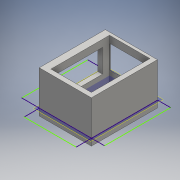
# Autodesk Inventor part: sampleHolderEnclosure
Saved by Autodesk Inventor 2016 (Build 200138000, 138)
## iProperties
Created: 2016-04-10
Part Number: sampleHolderEnclosure
Material: Generic
Document SubType Name: Modeling
Designer: sims01
Density: 1 g/cm^3
Appearance: Default
Author: sims01
Autodesk Inventor part; units mm, degrees
ref_plane "YZ Plane" through (0, 0, 0) normal (1, 0, 0) x (0, 1, 0)
ref_plane "XZ Plane" through (0, 0, 0) normal (0, 1, 0) x (-1, 0, 0)
ref_plane "XY Plane" through (0, 0, 0) normal (0, 0, 1) x (1, 0, 0)
sketch "Sketch1" plane through (0, 0, 0) normal (0, 0, 1) x (1, 0, 0)
  line L0 (-28, 35.5) -> (28, 35.5)
  line L1 (28, 35.5) -> (28, -35.5)
  line L2 (28, -35.5) -> (-28, -35.5)
  line L3 (-28, -35.5) -> (-28, 35.5)
  line L4 (-20.5, 32.5) -> (23, 32.5)
  line L5 (23, 32.5) -> (23, -30.5)
  line L6 (23, -30.5) -> (-20.5, -30.5)
  line L7 (-20.5, -30.5) -> (-20.5, 32.5)
  point P0 (0, 0)
  dimension "d0" = 56
  dimension "d1" = 28
  dimension "d2" = 71
  dimension "d3" = 35.5
  dimension "d4" = 3
  dimension "d5" = 7.5
  dimension "d7" = 5
  dimension "d8" = 5
  constraints: 16 end point, 4 parallel, 2 horizontal, 2 perpendicular
  measures "d0" distance of L0.start L0.end
  measures "d1" distance from line of point (0, 0) L1
  measures "d2" distance of L2.end L0.start
  measures "d3" distance from line of point (0, 0) L0
  measures "d4" distance between parallel lines of L4 L0
  measures "d5" distance between parallel lines of L3 L7
  measures "d7" distance between parallel lines of L2 L6
  measures "d8" distance between parallel lines of L1 L5
extrude "Extrusion1" add sketch "Sketch1" along normal blind 45
sketch "Sketch2" plane through (-28, -35.5, 0) normal (-1, 0, 0) x (0, 0, 1)
  line L0 (37.5, 60.5) -> (12.5, 60.5)
  line L1 (12.5, 60.5) -> (12.5, 10.5)
  line L2 (12.5, 10.5) -> (37.5, 10.5)
  line L3 (37.5, 10.5) -> (37.5, 60.5)
  point P0 (0, 35.5)
  dimension "d11" = 50
  dimension "d12" = 25
  dimension "d13" = 25
  dimension "d14" = 12.5
  constraints: 8 end point, 2 parallel, 1 horizontal, 1 perpendicular
  measures "d11" distance of L2.end L0.start
  measures "d12" distance from line of point (0, 35.5) L2
  measures "d13" distance of L1.end L2.end
  measures "d14" distance from line of point (0, 35.5) L1
extrude "Extrusion2" cut sketch "Sketch2" against normal up to surface (7.5 mm away)
sketch "Sketch4" plane through (-28, -35.5, 0) normal (-1, 0, 0) x (0, 0, 1)
  line L0 (40, 64.25) -> (10, 64.25)
  line L1 (10, 64.25) -> (10, 6.75)
  line L2 (10, 6.75) -> (40, 6.75)
  line L3 (40, 6.75) -> (40, 64.25)
  line L4 (0, 0) -> (0, 71) projected
  point P0 (0, 35.5)
  dimension "d23" = 57.5
  dimension "d24" = 30
  dimension "d25" = 28.75
  dimension "d26" = 10
  constraints: 8 end point, 2 parallel, 1 horizontal, 1 perpendicular
  measures "d23" distance of L2.end L0.start
  measures "d24" distance of L0.start L0.end
  measures "d25" distance from line of point (0, 35.5) L2
  measures "d26" distance between parallel lines of L4 L1
extrude "Extrusion4" cut sketch "Sketch4" against normal blind 2.5
sketch "Sketch5" plane through (-28, 35.5, 0) normal (0, 1, 0) x (1, 0, 0)
  line L0 (51.75, -40) -> (4.25, -40)
  line L1 (4.25, -40) -> (4.25, -10)
  line L2 (4.25, -10) -> (51.75, -10)
  line L3 (51.75, -10) -> (51.75, -40)
  line L4 (0, 0) -> (56, 0) projected
  point P0 (28, 0)
  dimension "d29" = 10
  dimension "d30" = 30
  dimension "d31" = 47.5
  dimension "d32" = 23.75
  constraints: 8 end point, 2 parallel, 1 horizontal, 1 perpendicular
  measures "d29" distance between parallel lines of L4 L2
  measures "d30" distance of L0.end L1.end
  measures "d31" distance of L0.start L0.end
  measures "d32" distance from line of L1 point (28, 0)
extrude "Extrusion5" cut sketch "Sketch5" against normal blind 2.5
sketch "Sketch6" plane through (-28, 35.5, 0) normal (0, 1, 0) x (1, 0, 0)
  line L0 (48, -37.5) -> (8, -37.5)
  line L1 (8, -37.5) -> (8, -12.5)
  line L2 (8, -12.5) -> (48, -12.5)
  line L3 (48, -12.5) -> (48, -37.5)
  point P0 (28, 0)
  dimension "d35" = 40
  dimension "d36" = 20
  dimension "d37" = 25
  dimension "d38" = 12.5
  constraints: 8 end point, 2 parallel, 1 horizontal, 1 perpendicular
  measures "d35" distance of L0.start L0.end
  measures "d36" distance from line of point (28, 0) L1
  measures "d37" distance of L2.end L0.start
  measures "d38" distance from line of point (28, 0) L2
extrude "Extrusion6" cut sketch "Sketch6" against normal up to surface (3 mm away)
ref_plane "Work Plane1" through (0, 0, 7.5) normal (0, 0, -1) x (-1, 0, 0)
sketch "Sketch8" plane through (0, 0, 7.5) normal (0, 0, -1) x (-1, 0, 0)
  line L0 (-42, 35.5) -> (-28, 35.5)
  line L1 (-28, 35.5) -> (-28, -35.5)
  line L2 (-28, -35.5) -> (-42, -35.5)
  line L3 (-42, -35.5) -> (-42, 35.5)
  line L4 (-28, -35.5) -> (28, -35.5)
  line L5 (28, -35.5) -> (28, -52)
  line L6 (28, -52) -> (-28, -52)
  line L7 (-28, -52) -> (-28, -35.5)
  line L8 (28, 35.5) -> (47, 35.5)
  line L9 (47, 35.5) -> (47, -35.5)
  line L10 (47, -35.5) -> (28, -35.5)
  line L11 (28, -35.5) -> (28, 35.5)
  line L12 (-28, 35.5) -> (28, 35.5) projected
  line L13 (28, -35.5) -> (-28, -35.5) projected
  line L14 (-28, -35.5) -> (-28, 35.5) projected
  line L15 (28, 35.5) -> (28, -35.5) projected
  point P0 (0, 0)
  constraints: 24 end point, 9 collinear, 6 parallel, 3 horizontal, 3 perpendicular
equation "\"d1\" = 0.5 * d0"
equation "\"d3\" = 0.5 * d2"
equation "\"d7\" = d8"
equation "\"d12\" = 0.5 * d11"
equation "\"d25\" = 0.5 * d23"
equation "\"d32\" = 0.5 * d31"
equation "\"d36\" = 0.5 * d35"
body "Solid1"
